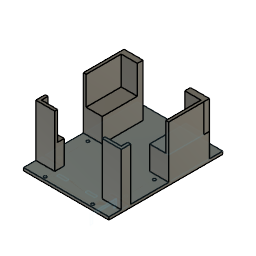
Robot base (Autodesk Fusion 360 design; units mm, degrees)
Autodesk Fusion 360 part; units mm, degrees
note: some values were not read from the file. Chosen so that the rebuilt part matches the saved one: which pieces of a blend or face edit are solid. Set by a fixed rule: the direction of a hole.
sketch "Sketch1" plane through (0, 0, 0) normal (0, 0, 1) x (1, 0, 0)
  line L0 (0, 0) -> (130, 0)
  line L1 (130, 0) -> (130, -120)
  line L2 (130, -120) -> (0, -120)
  line L3 (0, -120) -> (0, 0)
  dimension "d1" = 130
  dimension "d2" = 120
  constraint horizontal L0
  constraint vertical L1
  constraint horizontal L2
  constraint vertical L3
  constraint coincident L0.start L3.end
  measures "d1" distance of L0.start L0.end
  measures "d2" distance of L0.start L2.end
extrude "Extrude1" add sketch "Sketch1" along normal blind 3 makes body 1
sketch "Sketch2" plane through (0, 0, 0) normal (0, 0, 1) x (1, 0, 0)
  circle A0 centre (10, -10) radius 1.5
  line L0 (130, 0) -> (0, 0)
  line L1 (0, 0) -> (0, -120)
  circle A1 centre (10, -40) radius 1.5
  dimension "d5" = 3
  dimension "d6" = 10
  dimension "d7" = 10
  dimension "d8" = 3
  dimension "d9" = 10
  dimension "d10" = 30
  measures "d5" diameter of A0
  measures "d6" distance of A0.centre L0
  measures "d7" distance of A0.centre L1
  measures "d8" diameter of A1
  measures "d9" distance of L1 A1.centre
  measures "d10" distance of A0.centre A1.centre
hole "Hole1" at (10, -10, 0) at (10, -40, 0) direction (0, 0, 1) diameter 3 depth 16 tip angle 118 bodies 1
sketch "Sketch3" plane through (0, 0, 3) normal (0, 0, 1) x (-1, 0, 0)
  circle A0 centre (-10, 10) radius 1.5
  circle A1 centre (-10, 40) radius 1.5
  line L0 (0, 120) -> (-130, 120)
  line L1 (-130, 120) -> (-130, 0)
  line L2 (-130, 0) -> (0, 0)
  line L3 (0, 0) -> (0, 120)
  circle A2 centre (-120, 10) radius 1.5
  circle A3 centre (-120, 40) radius 1.5
  dimension "d14" = 3
  dimension "d15" = 3
  dimension "d16" = 10
  dimension "d17" = 10
  dimension "d18" = 30
  dimension "d19" = 10
  measures "d14" diameter of A2
  measures "d15" diameter of A3
  measures "d16" distance of L2 A2.centre
  measures "d17" distance of L1 A2.centre
  measures "d18" vertical distance of A2.centre A3.centre
  measures "d19" distance of L1 A3.centre
hole "Hole2" at (120, -10, 3) at (120, -40, 3) direction (0, 0, -1) diameter 3 depth 16 tip angle 118 bodies 1
sketch "Sketch4" plane through (0, 0, 3) normal (0, 0, 1) x (-1, 0, 0)
  circle A0 centre (-120, 10) radius 1.5
  circle A1 centre (-120, 40) radius 1.5
  circle A2 centre (-10, 10) radius 1.5
  circle A3 centre (-10, 40) radius 1.5
  line L0 (0, 120) -> (-130, 120)
  line L1 (-130, 120) -> (-130, 0)
  line L2 (-130, 0) -> (0, 0)
  line L3 (0, 0) -> (0, 120)
  line L4 (0, 120) -> (-65, 120) construction
  circle A4 centre (-40, 117) radius 1.5 construction
  line L5 (-65, 120) -> (-65, 112.4082) construction
  circle A5 centre (-90, 117) radius 1.5 construction
  dimension "d23" = 3
  dimension "d24" = 3
  dimension "d25" = 25
  dimension "d26" = 3
  dimension "d27" = 3
  dimension "d28" = 25
  constraint coincident L0.start L3.end
  constraint midpoint L0 L4.end
  constraint perpendicular L0 L5
  measures "d23" diameter of A4
  measures "d24" distance of L4 A4.centre
  measures "d25" distance of A4.centre L5
  measures "d26" diameter of A5
  measures "d27" distance of L0 A5.centre
  measures "d28" distance of L5 A5.centre
hole "Hole3" at (40, -117, 3) at (90, -117, 3) direction (0, 0, -1) diameter 3 depth 16 tip angle 118 bodies 1
sketch "Sketch5" plane through (0, 0, 0) normal (0, 1, 0) x (1, 0, 0)
ref_plane "WorkPlane1" through (65, -110, 1.5) normal (0, -1, 0) x (1, 0, 0)
sketch "Sketch6" plane through (0, -110, 0) normal (0, -1, 0) x (-1, 0, 0)
  line L0 (0, -3) -> (-65, -3) construction
  line L1 (-65, -3) -> (-55, -3)
  line L2 (-65, -3) -> (-75, -3)
  line L3 (-55, -3) -> (-45, -3)
  line L4 (-45, -3) -> (-45, -11)
  line L5 (-45, -11) -> (-55, -11)
  line L6 (-55, -11) -> (-55, -3)
  line L7 (-75, -3) -> (-85, -3)
  line L8 (-85, -3) -> (-85, -11)
  line L9 (-85, -11) -> (-75, -11)
  line L10 (-75, -11) -> (-75, -3)
  dimension "d33" = 65
  dimension "d34" = 10
  dimension "d35" = 10
  dimension "d36" = 10
  dimension "d37" = 8
  dimension "d38" = 10
  dimension "d39" = 8
  constraint horizontal L0
  constraint parallel L0 L1
  constraint parallel L1 L2
  constraint horizontal L3
  constraint vertical L4
  constraint horizontal L5
  constraint vertical L6
  constraint horizontal L7
  constraint vertical L8
  constraint horizontal L9
  constraint vertical L10
  measures "d33" distance of L0.start L0.end
  measures "d34" distance of L0.end L1.end
  measures "d35" distance of L0.end L2.end
  measures "d36" distance of L1.end L3.end
  measures "d37" distance of L1.end L5.end
  measures "d38" distance of L2.end L7.end
  measures "d39" distance of L2.end L9.end
extrude "Extrude2" add sketch "Sketch6" against normal blind 3 bodies 1
sketch "Sketch7" plane through (0, -110, 0) normal (0, -1, 0) x (1, 0, 0)
  line L0 (55, 11) -> (45, 11)
  line L1 (45, 11) -> (45, 3)
  line L2 (45, 3) -> (55, 3)
  line L3 (55, 3) -> (55, 11)
  line L4 (45, 11) -> (55, 11)
  line L5 (55, 11) -> (55, 8)
  line L6 (55, 8) -> (45, 8)
  line L7 (45, 8) -> (45, 11)
  line L8 (75, 11) -> (85, 11)
  line L9 (85, 11) -> (85, 8)
  line L10 (85, 8) -> (75, 8)
  line L11 (75, 8) -> (75, 11)
  dimension "d42" = 10
  dimension "d43" = 3
  dimension "d44" = 10
  dimension "d45" = 3
  constraint horizontal L4
  constraint vertical L5
  constraint horizontal L6
  constraint vertical L7
  constraint coincident L0.end L1.start
  constraint horizontal L8
  constraint vertical L9
  constraint horizontal L10
  constraint vertical L11
  measures "d42" distance of L0.end L0.start
  measures "d43" distance of L0.end L6.end
  measures "d44" distance of L8.start L8.end
  measures "d45" distance of L8.start L10.end
extrude "Extrude3" add sketch "Sketch7" along normal blind 25 contours L0 L1 L3 L4 L5 L6 L7 | L8 L9 L10 L11 bodies 1
sketch "Sketch8" plane through (0, 0, 8) normal (0, 0, -1) x (1, 0, 0)
  line L0 (45, 110) -> (55, 110)
  line L1 (55, 110) -> (55, 135)
  line L2 (55, 135) -> (45, 135)
  line L3 (45, 135) -> (45, 110)
  line L4 (45, 135) -> (55, 135)
  line L5 (55, 135) -> (55, 132)
  line L6 (55, 132) -> (45, 132)
  line L7 (45, 132) -> (45, 135)
  line L8 (75, 135) -> (85, 135)
  line L9 (85, 135) -> (85, 132)
  line L10 (85, 132) -> (75, 132)
  line L11 (75, 132) -> (75, 135)
  dimension "d48" = 10
  dimension "d49" = 3
  dimension "d50" = 10
  dimension "d51" = 3
  constraint horizontal L4
  constraint vertical L5
  constraint horizontal L6
  constraint vertical L7
  constraint coincident L2.end L3.start
  constraint horizontal L8
  constraint vertical L9
  constraint horizontal L10
  constraint vertical L11
  measures "d48" distance of L2.end L1.end
  measures "d49" distance of L2.end L6.end
  measures "d50" distance of L8.start L8.end
  measures "d51" distance of L8.start L10.end
extrude "Extrude4" add sketch "Sketch8" along normal blind 8 contours L1 L2 L3 L4 L5 L6 L7 | L8 L9 L10 L11 bodies 1
sketch "Sketch9" plane through (85, 0, 0) normal (1, 0, 0) x (0, 1, 0)
  line L0 (-110, 8) -> (-110, 3)
  line L1 (-110, 3) -> (-107, 3)
  line L2 (-107, 3) -> (-107, 11)
  line L3 (-107, 11) -> (-135, 11)
  line L4 (-135, 11) -> (-135, 0)
  line L5 (-135, 0) -> (-132, 0)
  line L6 (-132, 0) -> (-132, 8)
  line L7 (-132, 8) -> (-110, 8)
sketch "Sketch10" plane through (0, -135, 0) normal (0, -1, 0) x (1, 0, 0)
  line L0 (85, 0) -> (85, 11)
  line L1 (85, 11) -> (75, 11)
  line L2 (75, 11) -> (75, 0)
  line L3 (75, 0) -> (85, 0)
  line L4 (0, 0) -> (65, 0) construction
  line L5 (65, 0) -> (40, 0)
  line L6 (65, 0) -> (90, 0)
  line L7 (40, 0) -> (40, 60)
  line L8 (40, 60) -> (90, 60)
  line L9 (90, 60) -> (90, 0)
  dimension "d54" = 65
  dimension "d55" = 25
  dimension "d56" = 25
  dimension "d57" = 60
  dimension "d58" = 50
  constraint coincident L4.start origin
  constraint horizontal L4
  constraint parallel L4 L5
  constraint parallel L3 L6
  constraint perpendicular L4 L7
  constraint perpendicular L7 L8
  measures "d54" distance of L4.start L4.end
  measures "d55" distance of L4.end L5.end
  measures "d56" distance of L4.end L6.end
  measures "d57" distance of L5.end L7.end
  measures "d58" distance of L7.end L8.end
extrude "Extrude5" add sketch "Sketch10" against normal blind 3 contours L0 L1 L2 L5 L6 L7 L8 L9 bodies 1
sketch "Sketch12" plane through (0, 0, 3) normal (0, 0, 1) x (-1, 0, 0)
  line L0 (0, 50) -> (-20, 50)
  line L1 (-20, 50) -> (0, 50)
  line L2 (0, 50) -> (0, 120)
  line L3 (0, 120) -> (-20, 120)
  line L4 (-20, 120) -> (-20, 50)
  dimension "d62" = 20
  constraint horizontal L0
  constraint horizontal L1
  constraint vertical L2
  constraint horizontal L3
  constraint vertical L4
  measures "d62" distance of L0.start L0.end
sketch "Sketch13" plane through (0, 0, 3) normal (0, 0, 1) x (-1, 0, 0)
  line L0 (-130, 120) -> (-110, 120)
  line L1 (-110, 120) -> (-110, 50)
  line L2 (-110, 50) -> (-130, 50)
  line L3 (-130, 50) -> (-130, 120)
  dimension "d63" = 20
  dimension "d64" = 70
  constraint horizontal L0
  constraint vertical L1
  constraint horizontal L2
  constraint vertical L3
  measures "d63" distance of L0.start L0.end
  measures "d64" distance of L0.start L2.end
extrude "Extrude6" cut sketch "Sketch12" sketch "Sketch13" against normal blind 15 of sketch 2 bodies 1
fillet "Fillet1" radius 20 1 edges at (20, -50, 1.5) on bodies 1
fillet "Fillet2" radius 20 1 edges at (110, -50, 1.5) on bodies 1
sketch "Sketch14" plane through (0, 0, 3) normal (0, 0, 1) x (-1, 0, 0)
  line L0 (-20, 70) -> (-20, 120)
  line L1 (-20, 120) -> (-110, 120)
  line L2 (-110, 120) -> (-110, 70)
  arc A0 (-130, 50) -> (-110, 70) centre (-130, 70) ccw
  line L3 (-130, 50) -> (-130, 0)
  line L4 (-130, 0) -> (0, 0)
  line L5 (0, 0) -> (0, 50)
  arc A1 (-20, 70) -> (0, 50) centre (0, 70) ccw
  line L6 (-75, 110) -> (-75, 107)
  line L7 (-75, 107) -> (-85, 107)
  line L8 (-85, 107) -> (-85, 110)
  line L9 (-85, 110) -> (-75, 110)
  line L10 (-55, 107) -> (-55, 110)
  line L11 (-55, 110) -> (-45, 110)
  line L12 (-45, 110) -> (-45, 107)
  line L13 (-45, 107) -> (-55, 107)
  circle A2 centre (-40, 117) radius 1.5
  circle A3 centre (-90, 117) radius 1.5
  circle A4 centre (-120, 10) radius 1.5
  circle A5 centre (-120, 40) radius 1.5
  circle A6 centre (-10, 10) radius 1.5
  circle A7 centre (-10, 40) radius 1.5
  circle A8 centre (-30, 70) radius 1.5
  circle A9 centre (-30, 100) radius 1.5
  dimension "d71" = 3
  dimension "d72" = 3
  dimension "d73" = 10
  dimension "d74" = 10
  dimension "d75" = 30
  dimension "d76" = 20
  measures "d71" diameter of A8
  measures "d72" diameter of A9
  measures "d73" distance of L0 A8.centre
  measures "d74" distance of L0 A9.centre
  measures "d75" distance of A8.centre A9.centre
  measures "d76" distance of L1 A9.centre
sketch "Sketch15" plane through (0, 0, 3) normal (0, 0, 1) x (1, 0, 0)
  circle A0 centre (100, -70) radius 1.5
  circle A1 centre (100, -100) radius 1.5
  line L0 (110, -120) -> (110, -70)
  line L1 (0, -120) -> (130, -120)
  point P0 (110, -70)
  dimension "d77" = 3
  dimension "d78" = 3
  dimension "d79" = 30
  dimension "d80" = 10
  dimension "d81" = 10
  dimension "d82" = 20
  measures "d77" diameter of A0
  measures "d78" diameter of A1
  measures "d79" distance of A0.centre A1.centre
  measures "d80" distance of A0.centre P0
  measures "d81" distance of A1.centre L0
  measures "d82" distance of A1.centre L1
hole "Hole4" at (30, -70, 3) at (30, -100, 3) at (100, -70, 3) at (100, -100, 3) direction (0, 0, -1) diameter 3 depth 16 tip angle 118 bodies 1
sketch "Sketch16" plane through (0, 0, 3) normal (0, 0, 1) x (-1, 0, 0)
  line L0 (0, 0) -> (-20, 0)
  line L1 (-20, 0) -> (-20, 70)
  line L2 (-20, 70) -> (0, 70)
  line L3 (0, 70) -> (0, 0)
  line L4 (-130, 0) -> (-110, 0)
  line L5 (-110, 0) -> (-110, 70)
  line L6 (-110, 70) -> (-130, 70)
  line L7 (-130, 70) -> (-130, 0)
  constraint horizontal L0
  constraint vertical L1
  constraint horizontal L2
  constraint vertical L3
  constraint coincident L0.start L3.end
  constraint horizontal L4
  constraint vertical L5
  constraint horizontal L6
  constraint vertical L7
extrude "Extrude7" cut sketch "Sketch16" against normal blind 25 bodies 1
sketch "Sketch17" plane through (0, -135, 0) normal (0, -1, 0) x (1, 0, 0)
  line L0 (40, 0) -> (90, 0)
  line L1 (90, 0) -> (90, 60)
  line L2 (90, 60) -> (40, 60)
  line L3 (40, 60) -> (40, 0)
extrude "Extrude8" cut sketch "Sketch17" against normal blind 3 bodies 1
sketch "Sketch18" plane through (0, 0, 0) normal (0, 0, 1) x (1, 0, 0)
  line L0 (0, 0) -> (-85, 0)
  line L1 (-85, 0) -> (-85, 80)
  line L2 (-85, 80) -> (0, 80)
  line L3 (0, 80) -> (0, 0)
  dimension "d90" = 85
  dimension "d91" = 80
  constraint horizontal L0
  constraint vertical L1
  constraint horizontal L2
  constraint vertical L3
  constraint coincident L0.start L3.end
  measures "d90" distance of L0.start L0.end
  measures "d91" distance of L0.start L2.end
extrude "Extrude9" add sketch "Sketch18" along normal blind 20 separate body makes body 2
move_body "Move1" bodies 2 to x (1, 0, 0) y (0, 1, 0) z (0, 0, 1) at (90, 0, 3)
move_body "Move2" bodies 2 to x (1, 0, 0) y (0, 1, 0) z (0, 0, 1) at (17.5, -80, 0)
move_body "Move3" bodies 2 to x (1, 0, 0) y (0, 1, 0) z (0, 0, 1) at (0, 15, 0)
move_body "Move4" bodies 2 to x (0, 1, 0) y (-1, 0, 0) z (0, 0, 1) at (0, 0, 0)
sketch "Sketch19" plane through (0, 0, 3) normal (0, 0, 1) x (-1, 0, 0)
sketch "Sketch20" plane through (0, 0, 3) normal (0, 0, 1) x (-1, 0, 0)
sketch "Sketch21" plane through (0, 0, 3) normal (0, 0, 1) x (-1, 0, 0)
  line L0 (-110, 120) -> (-110, 0)
  line L1 (-110, 0) -> (-20, 0)
  line L2 (-20, 0) -> (-20, 120)
  line L3 (-20, 120) -> (-110, 120)
  circle A0 centre (-100, 70) radius 1.5
  circle A1 centre (-30, 70) radius 1.5
  circle A2 centre (-30, 100) radius 1.5
  circle A3 centre (-100, 100) radius 1.5
  line L4 (-75, 110) -> (-75, 107)
  line L5 (-75, 107) -> (-85, 107)
  line L6 (-85, 107) -> (-85, 110)
  line L7 (-85, 110) -> (-75, 110)
  line L8 (-55, 107) -> (-55, 110)
  line L9 (-55, 110) -> (-45, 110)
  line L10 (-45, 110) -> (-45, 107)
  line L11 (-45, 107) -> (-55, 107)
  circle A4 centre (-40, 117) radius 1.5
  circle A5 centre (-90, 117) radius 1.5
  line L12 (-20, 67.4975) -> (-110, 67.4975)
  line L13 (-110, 67.4975) -> (-110, 105)
  line L14 (-110, 105) -> (-20, 105)
  line L15 (-20, 105) -> (-20, 67.4975)
  constraint horizontal L12
  constraint vertical L13
  constraint horizontal L14
  constraint vertical L15
  constraint coincident L0 L13.end
  constraint coincident L2 L12.start
extrude "Extrude10" add sketch "Sketch21" against normal blind 3 contours A0 | A1 | A2 | A3 bodies 1
sketch "Sketch22" plane through (0, 0, 3) normal (0, 0, 1) x (-1, 0, 0)
  line L0 (-110, 120) -> (-110, 0)
  line L1 (-110, 0) -> (-20, 0)
  line L2 (-20, 0) -> (-20, 120)
  line L3 (-20, 120) -> (-110, 120)
  line L4 (-75, 110) -> (-75, 107)
  line L5 (-75, 107) -> (-85, 107)
  line L6 (-85, 107) -> (-85, 110)
  line L7 (-85, 110) -> (-75, 110)
  line L8 (-55, 107) -> (-55, 110)
  line L9 (-55, 110) -> (-45, 110)
  line L10 (-45, 110) -> (-45, 107)
  line L11 (-45, 107) -> (-55, 107)
  circle A0 centre (-40, 117) radius 1.5
  circle A1 centre (-90, 117) radius 1.5
  line L12 (-20, 120) -> (-20, 100) construction
  line L13 (-20, 100) -> (-40, 100)
  line L14 (-40, 100) -> (-40, 97)
  line L15 (-40, 97) -> (-20, 97)
  line L16 (-20, 97) -> (-20, 100)
  line L17 (-20, 97) -> (-20, 57) construction
  line L18 (-20, 57) -> (-40, 57)
  line L19 (-40, 57) -> (-40, 54)
  line L20 (-40, 54) -> (-20, 54)
  line L21 (-20, 54) -> (-20, 57)
  dimension "d97" = 20
  dimension "d98" = 3
  dimension "d99" = 40
  dimension "d100" = 20
  dimension "d101" = 3
  constraint coincident L2.end L3.start
  constraint coincident L2 L12.end
  constraint horizontal L13
  constraint vertical L14
  constraint horizontal L15
  constraint vertical L16
  constraint perpendicular L15 L17
  constraint horizontal L18
  constraint vertical L19
  constraint horizontal L20
  constraint vertical L21
  measures "d97" distance of L12.end L13.end
  measures "d98" distance of L12.end L15.end
  measures "d99" distance of L15.end L17.end
  measures "d100" distance of L17.end L18.end
  measures "d101" distance of L17.end L20.end
extrude "Extrude11" add sketch "Sketch22" along normal blind 28 contours L2 L13 L14 L15 L16 | L2 L18 L19 L20 L21 bodies 1
sketch "Sketch23" plane through (0, -97, 0) normal (0, 1, 0) x (-1, 0, 0)
  line L0 (-40, 3) -> (-20, 3)
  line L1 (-20, 3) -> (-20, 31)
  line L2 (-20, 31) -> (-40, 31)
  line L3 (-40, 31) -> (-40, 3)
  line L4 (-40, 31) -> (-20, 31)
  line L5 (-20, 31) -> (-20, 28)
  line L6 (-20, 28) -> (-40, 28)
  line L7 (-40, 28) -> (-40, 31)
  dimension "d104" = 20
  dimension "d105" = 3
  constraint horizontal L4
  constraint vertical L5
  constraint horizontal L6
  constraint vertical L7
  constraint coincident L2.end L3.start
  measures "d104" distance of L2.end L1.end
  measures "d105" distance of L2.end L6.end
extrude "Extrude12" add sketch "Sketch23" along normal blind 40 contours L1 L2 L3 L4 L5 L6 L7 bodies 1
move_body "Move5" bodies 1 to x (1, 0, 0) y (0, 1, 0) z (0, 0, 1) at (-20, 0, 0)
ref_plane "WorkPlane2" through (45, 0, 0) normal (1, 0, 0) x (0, 1, 0)
mirror "Mirror1" about plane through (45, 0, 0) normal (1, 0, 0) of bodies 1 merged
sketch "Sketch24" plane through (0, 0, 3) normal (0, 0, 1) x (-1, 0, 0)
  circle A0 centre (-70, 117) radius 1.5
  circle A1 centre (-20, 117) radius 1.5
  line L0 (-35, 107) -> (-35, 110)
  line L1 (-35, 110) -> (-25, 110)
  line L2 (-25, 110) -> (-25, 107)
  line L3 (-25, 107) -> (-35, 107)
  line L4 (-55, 110) -> (-55, 107)
  line L5 (-55, 107) -> (-65, 107)
  line L6 (-65, 107) -> (-65, 110)
  line L7 (-65, 110) -> (-55, 110)
  line L8 (-90, 100) -> (-70, 100)
  line L9 (-70, 100) -> (-70, 97)
  line L10 (-70, 97) -> (-90, 97)
  line L11 (-90, 97) -> (-90, 57)
  line L12 (-90, 57) -> (-70, 57)
  line L13 (-70, 57) -> (-70, 54)
  line L14 (-70, 54) -> (-90, 54)
  line L15 (-90, 54) -> (-90, 0)
  line L16 (-90, 0) -> (0, 0)
  line L17 (0, 0) -> (0, 54)
  line L18 (0, 54) -> (-20, 54)
  line L19 (-20, 54) -> (-20, 57)
  line L20 (-20, 57) -> (0, 57)
  line L21 (0, 57) -> (0, 97)
  line L22 (0, 97) -> (-20, 97)
  line L23 (-20, 97) -> (-20, 100)
  line L24 (-20, 100) -> (0, 100)
  line L25 (0, 100) -> (0, 120)
  line L26 (0, 120) -> (-90, 120)
  line L27 (-90, 120) -> (-90, 100)
  circle A2 centre (-10, 62) radius 1.5
  circle A3 centre (-10, 92) radius 1.5
  circle A4 centre (-79.3254, 63.9731) radius 1.5
  circle A5 centre (-81.7658, 88.1327) radius 1.5
  dimension "d111" = 3
  dimension "d112" = 3
  dimension "d113" = 3
  dimension "d114" = 3
  dimension "d115" = 10
  dimension "d116" = 10
  dimension "d117" = 30
  dimension "d118" = 5
  measures "d111" diameter of A2
  measures "d112" diameter of A3
  measures "d113" diameter of A4
  measures "d114" diameter of A5
  measures "d115" distance of L21 A3.centre
  measures "d116" distance of L21 A2.centre
  measures "d117" distance of A2.centre A3.centre
  measures "d118" distance of L20 A2.centre
hole "Hole5" at (10, -62, 3) at (10, -92, 3) direction (0, 0, -1) diameter 3 depth 16 tip angle 118 bodies 1
sketch "Sketch25" plane through (0, 0, 3) normal (0, 0, 1) x (-1, 0, 0)
  circle A0 centre (-10, 62) radius 1.5
  circle A1 centre (-10, 92) radius 1.5
  circle A2 centre (-70, 117) radius 1.5
  circle A3 centre (-20, 117) radius 1.5
  line L0 (-35, 107) -> (-35, 110)
  line L1 (-35, 110) -> (-25, 110)
  line L2 (-25, 110) -> (-25, 107)
  line L3 (-25, 107) -> (-35, 107)
  line L4 (-55, 110) -> (-55, 107)
  line L5 (-55, 107) -> (-65, 107)
  line L6 (-65, 107) -> (-65, 110)
  line L7 (-65, 110) -> (-55, 110)
  line L8 (-90, 100) -> (-70, 100)
  line L9 (-70, 100) -> (-70, 97)
  line L10 (-70, 97) -> (-90, 97)
  line L11 (-90, 97) -> (-90, 57)
  line L12 (-90, 57) -> (-70, 57)
  line L13 (-70, 57) -> (-70, 54)
  line L14 (-70, 54) -> (-90, 54)
  line L15 (-90, 54) -> (-90, 0)
  line L16 (-90, 0) -> (0, 0)
  line L17 (0, 0) -> (0, 54)
  line L18 (0, 54) -> (-20, 54)
  line L19 (-20, 54) -> (-20, 57)
  line L20 (-20, 57) -> (0, 57)
  line L21 (0, 57) -> (0, 97)
  line L22 (0, 97) -> (-20, 97)
  line L23 (-20, 97) -> (-20, 100)
  line L24 (-20, 100) -> (0, 100)
  line L25 (0, 100) -> (0, 120)
  line L26 (0, 120) -> (-90, 120)
  line L27 (-90, 120) -> (-90, 100)
  circle A4 centre (-80, 62) radius 1.5
  circle A5 centre (-80, 92) radius 1.5
  dimension "d122" = 3
  dimension "d123" = 3
  dimension "d124" = 10
  dimension "d125" = 10
  dimension "d126" = 30
  dimension "d127" = 5
  measures "d122" diameter of A4
  measures "d123" diameter of A5
  measures "d124" distance of L11 A4.centre
  measures "d125" distance of L11 A5.centre
  measures "d126" distance of A4.centre A5.centre
  measures "d127" distance of L12 A4.centre
hole "Hole6" at (80, -62, 3) at (80, -92, 3) direction (0, 0, -1) diameter 3 depth 16 tip angle 118 bodies 1
sketch "Sketch26" plane through (0, 0, 31) normal (0, 0, 1) x (-1, 0, 0)
  line L0 (-90, 100) -> (-90, 54)
  line L1 (-90, 54) -> (-70, 54)
  line L2 (-70, 54) -> (-70, 100)
  line L3 (-70, 100) -> (-90, 100)
  line L4 (0, 54) -> (-90, 54)
  line L5 (-90, 54) -> (-90, 100)
  line L6 (-90, 100) -> (0, 100)
  line L7 (0, 100) -> (0, 54)
  constraint horizontal L4
  constraint vertical L5
  constraint horizontal L6
  constraint vertical L7
  constraint coincident L0.start L3.end
extrude "Extrude13" cut sketch "Sketch26" against normal blind 3 bodies 1
move_body "Move6" bodies 2 to x (1, 0, 0) y (0, 1, 0) z (0, 0, 1) at (25, -122.5, 25)
sketch "Sketch27" plane through (0, 0, 3) normal (0, 0, 1) x (-1, 0, 0)
  circle A0 centre (-80, 62) radius 1.5
  circle A1 centre (-80, 92) radius 1.5
  circle A2 centre (-10, 62) radius 1.5
  circle A3 centre (-10, 92) radius 1.5
  circle A4 centre (-70, 117) radius 1.5
  circle A5 centre (-20, 117) radius 1.5
  line L0 (-35, 107) -> (-35, 110)
  line L1 (-35, 110) -> (-25, 110)
  line L2 (-25, 110) -> (-25, 107)
  line L3 (-25, 107) -> (-35, 107)
  line L4 (-55, 110) -> (-55, 107)
  line L5 (-55, 107) -> (-65, 107)
  line L6 (-65, 107) -> (-65, 110)
  line L7 (-65, 110) -> (-55, 110)
  line L8 (-90, 100) -> (-70, 100)
  line L9 (-70, 100) -> (-70, 97)
  line L10 (-70, 97) -> (-90, 97)
  line L11 (-90, 97) -> (-90, 57)
  line L12 (-90, 57) -> (-70, 57)
  line L13 (-70, 57) -> (-70, 54)
  line L14 (-70, 54) -> (-90, 54)
  line L15 (-90, 54) -> (-90, 0)
  line L16 (-90, 0) -> (0, 0)
  line L17 (0, 0) -> (0, 54)
  line L18 (0, 54) -> (-20, 54)
  line L19 (-20, 54) -> (-20, 57)
  line L20 (-20, 57) -> (0, 57)
  line L21 (0, 57) -> (0, 97)
  line L22 (0, 97) -> (-20, 97)
  line L23 (-20, 97) -> (-20, 100)
  line L24 (-20, 100) -> (0, 100)
  line L25 (0, 100) -> (0, 120)
  line L26 (0, 120) -> (-90, 120)
  line L27 (-90, 120) -> (-90, 100)
extrude "Extrude14" add 1 faces at (6.6667, -100, 11.3333) along direction (0, -1, 0) blind 7 on bodies 1 bodies 1 2
move_face "MoveFace1" by (0, 0, 95) 1 faces at (56.6667, -100, 41.3333) on bodies 1
move_face "MoveFace2" by (0, 0, 25) 1 faces at (56.6667, -100, 41.3333) on bodies 1
delete_face "DeleteFace1" 1 faces at (56.6667, -100, 41.3333) on bodies 1
sketch "Sketch29" plane through (0, 0, 3) normal (0, 0, 1) x (1, 0, 0)
  line L0 (70.0558, -97) -> (90, -97)
  line L1 (90, -97) -> (90, -107)
  line L2 (90, -107) -> (70.0558, -107)
  line L3 (70.0558, -107) -> (70.0558, -97)
  constraint horizontal L0
  constraint vertical L1
  constraint horizontal L2
  constraint vertical L3
extrude "Extrude15" add sketch "Sketch29" along normal blind 35 bodies 1
extrude "Extrude16" cut 1 faces at (76.7038, -100.3333, 38) along direction (0, 0, -1) blind 10 on bodies 1 bodies 1
extrude "Extrude17" add 1 faces at (13.3333, -54, 19.6667) along direction (0, 1, 0) blind 15 on bodies 1 bodies 1
extrude "Extrude18" add 1 faces at (76.6667, -54, 11.3333) along direction (0, 1, 0) blind 15 on bodies 1 bodies 1
sketch "Sketch30" plane through (0, 0, 28) normal (0, 0, 1) x (-1, 0, 0)
  line L0 (-20, 97) -> (0, 97)
  line L1 (0, 97) -> (0, 107)
  line L2 (0, 107) -> (-20, 107)
  line L3 (-20, 107) -> (-20, 97)
  line L4 (0, 107) -> (-20, 107)
  line L5 (-20, 107) -> (-20, 104)
  line L6 (-20, 104) -> (0, 104)
  line L7 (0, 104) -> (0, 107)
  dimension "d143" = 3
  constraint horizontal L4
  constraint vertical L5
  constraint horizontal L6
  constraint vertical L7
  constraint coincident L1.end L2.start
  measures "d143" distance of L1.end L6.end
extrude "Extrude19" add sketch "Sketch30" along normal blind 30 contours L1 L2 L3 L4 L5 L6 L7 bodies 1
sketch "Sketch31" plane through (0, 0, 28) normal (0, 0, 1) x (-1, 0, 0)
  line L0 (0, 104) -> (-20, 104)
  line L1 (-20, 104) -> (-20, 97)
  line L2 (-20, 97) -> (0, 97)
  line L3 (0, 97) -> (0, 104)
  line L4 (0, 97) -> (-3, 97)
  line L5 (-3, 97) -> (-3, 104)
  line L6 (-3, 104) -> (0, 104)
  line L7 (0, 104) -> (0, 97)
  dimension "d146" = 3
  constraint horizontal L4
  constraint vertical L5
  constraint horizontal L6
  constraint vertical L7
  constraint coincident L2.end L3.start
  measures "d146" distance of L2.end L4.end
extrude "Extrude20" add sketch "Sketch31" along normal blind 30 contours L0 L2 L3 L4 L5 L6 L7 bodies 1
sketch "Sketch32" plane through (0, 0, 28) normal (0, 0, 1) x (-1, 0, 0)
  line L0 (-70.0558, 107) -> (-90, 107)
  line L1 (-90, 107) -> (-90, 97)
  line L2 (-90, 97) -> (-70.0558, 97)
  line L3 (-70.0558, 97) -> (-70.0558, 107)
  line L4 (-90, 107) -> (-70, 107)
  line L5 (-70, 107) -> (-70, 104)
  line L6 (-70, 104) -> (-90, 104)
  line L7 (-90, 104) -> (-90, 107)
  dimension "d149" = 20
  dimension "d150" = 3
  constraint horizontal L4
  constraint vertical L5
  constraint horizontal L6
  constraint vertical L7
  constraint coincident L0.end L1.start
  measures "d149" distance of L0.end L4.end
  measures "d150" distance of L0.end L6.end
extrude "Extrude21" add sketch "Sketch32" along normal blind 30 contours L0 L1 L3 L4 L6 L7 bodies 1
sketch "Sketch33" plane through (0, 0, 28) normal (0, 0, 1) x (-1, 0, 0)
  line L0 (-70.0558, 104) -> (-90, 104)
  line L1 (-90, 104) -> (-90, 97)
  line L2 (-90, 97) -> (-70.0558, 97)
  line L3 (-70.0558, 97) -> (-70.0558, 104)
  line L4 (-90, 104) -> (-87, 104)
  line L5 (-87, 104) -> (-87, 97)
  line L6 (-87, 97) -> (-90, 97)
  line L7 (-90, 97) -> (-90, 104)
  constraint horizontal L4
  constraint vertical L5
  constraint horizontal L6
  constraint vertical L7
  constraint coincident L2 L5.end
  constraint coincident L0.end L1.start
extrude "Extrude22" add sketch "Sketch33" along normal blind 30 contours L0 L1 L2 L4 L5 L6 L7 bodies 1
extrude "Extrude23" add 1 faces at (76.6667, -39, 11.3333) along direction (0, 1, 0) blind 20 on bodies 1 bodies 1
extrude "Extrude24" add 1 faces at (13.3333, -39, 19.6667) along direction (0, 1, 0) blind 20 on bodies 1 bodies 1
sketch "Sketch34" plane through (0, 0, 28) normal (0, 0, 1) x (-1, 0, 0)
  line L0 (-70, 57) -> (-90, 57)
  line L1 (-90, 57) -> (-90, 19)
  line L2 (-90, 19) -> (-70, 19)
  line L3 (-70, 19) -> (-70, 57)
extrude "Extrude25" add 1 faces at (76.6667, -19, 11.3333) along direction (0, 1, 0) blind 5 on bodies 1 bodies 1
extrude "Extrude26" add 1 faces at (13.3333, -19, 19.6667) along direction (0, 1, 0) blind 5 on bodies 1 bodies 1
sketch "Sketch35" plane through (0, 0, 28) normal (0, 0, 1) x (-1, 0, 0)
  line L0 (-90.0311, 14.0274) -> (-69.9996, 14.0274)
  line L1 (-69.9996, 14.0274) -> (-69.9996, 21.0274)
  line L2 (-69.9996, 21.0274) -> (-90.0311, 21.0274)
  line L3 (-90.0311, 21.0274) -> (-90.0311, 14.0274)
  dimension "d163" = 7
  constraint horizontal L0
  constraint vertical L1
  constraint horizontal L2
  constraint vertical L3
  measures "d163" distance of L0.start L2.end
extrude "Extrude27" add sketch "Sketch35" along normal blind 30 bodies 1
sketch "Sketch36" plane through (0, 0, 28) normal (0, 0, 1) x (-1, 0, 0)
  line L0 (0, 57) -> (-20, 57)
  line L1 (-20, 57) -> (-20, 14)
  line L2 (-20, 14) -> (0, 14)
  line L3 (0, 14) -> (0, 57)
  line L4 (0, 14) -> (-20, 14)
  line L5 (-20, 14) -> (-20, 21)
  line L6 (-20, 21) -> (0, 21)
  line L7 (0, 21) -> (0, 14)
  dimension "d166" = 7
  constraint horizontal L4
  constraint vertical L5
  constraint horizontal L6
  constraint vertical L7
  constraint coincident L1 L5.end
  constraint coincident L2.end L3.start
  measures "d166" distance of L2.end L6.end
extrude "Extrude28" add sketch "Sketch36" along normal blind 30 contours L1 L2 L3 L4 L5 L6 L7 bodies 1
extrude "Extrude29" cut 1 faces at (83.3436, -21.0274, 48) along direction (0, 1, 0) blind 1 on bodies 1 bodies 1
extrude "Extrude30" cut 1 faces at (13.3333, -21, 38) along direction (0, 1, 0) blind 1 on bodies 1 bodies 1
sketch "Sketch37" plane through (0, 0, 28) normal (0, 0, 1) x (-1, 0, 0)
  line L0 (0, 20) -> (-3, 20)
  line L1 (-3, 20) -> (-3, 57)
  line L2 (-3, 57) -> (0, 57)
  line L3 (0, 57) -> (0, 20)
  dimension "d173" = 3
  dimension "d174" = 37
  constraint horizontal L0
  constraint vertical L1
  constraint horizontal L2
  constraint vertical L3
  measures "d173" distance of L0.start L0.end
  measures "d174" distance of L0.start L2.end
extrude "Extrude31" add sketch "Sketch37" along normal blind 30 bodies 1
sketch "Sketch38" plane through (0, 0, 28) normal (0, 0, 1) x (-1, 0, 0)
sketch "Sketch39" plane through (0, 0, 28) normal (0, 0, 1) x (-1, 0, 0)
  line L0 (-90, 57) -> (-87, 57)
  line L1 (-87, 57) -> (-87, 20)
  line L2 (-87, 20) -> (-90, 20)
  line L3 (-90, 20) -> (-90, 57)
  dimension "d177" = 3
  dimension "d178" = 37
  constraint horizontal L0
  constraint vertical L1
  constraint horizontal L2
  constraint vertical L3
  measures "d177" distance of L0.start L0.end
  measures "d178" distance of L0.start L2.end
extrude "Extrude32" add sketch "Sketch39" along normal blind 30 bodies 1
sketch "Sketch40" plane through (0, 0, 11) normal (0, 0, 1) x (-1, 0, 0)
  line L0 (-25, 132) -> (-35, 132)
  line L1 (-35, 132) -> (-35, 107)
  line L2 (-35, 107) -> (-25, 107)
  line L3 (-25, 107) -> (-25, 132)
  line L4 (-25, 107) -> (-65, 107)
  line L5 (-65, 107) -> (-65, 132)
  line L6 (-65, 132) -> (-25, 132)
  line L7 (-25, 132) -> (-25, 107)
  constraint horizontal L4
  constraint vertical L5
  constraint horizontal L6
  constraint vertical L7
  constraint coincident L2.end L3.start
extrude "Extrude33" cut sketch "Sketch40" against normal blind 8 bodies 1
sketch "Sketch41" plane through (0, 0, 58) normal (0, 0, 1) x (-1, 0, 0)
  line L0 (-70.0558, 104) -> (-70.0558, 107)
  line L1 (-70.0558, 107) -> (-90, 107)
  line L2 (-90, 107) -> (-90, 97)
  line L3 (-90, 97) -> (-87, 97)
  line L4 (-87, 97) -> (-87, 104)
  line L5 (-87, 104) -> (-70.0558, 104)
